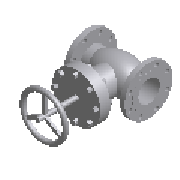
# Autodesk Inventor part: ASME B16.34 Globe Valve Flanged Ends - Class 150 8
Saved by Autodesk Inventor 2019.1 (Build 231200000, 200)
## iProperties
Created: 2018-01-05
Part Number: ASME B16.34 Globe Valve Flanged Ends - Class 150 8
Material: Steel
Description: Globe Valve
Document SubType Name: Modeling
Standard: ASME B16.34
Designer: alid
Standards Organization: ANSI
Language: en-US
Size Designation: 8
Categories: <MemberInstance><Categories><Category DisplayName="Tube &amp; Pipe" InternalName="4347fa0f-2144-441d-94cd-e3e15c92b736" Mnemonic="TUBEANDPIPE"><CategoryParameter DisplayName="Number of Connections" InternalName="04e9c83a-9e20-4a98-a7e1-e8abe87a2846" Mnemonic="NUM_CONNECTIONS"/><CategoryParameter DisplayName="Angles" InternalName="0e0e4fa4-3bd3-4656-a22e-4e07c8c476f8" Mnemonic="ANGLES"><CategoryParameter DisplayName="Angle" InternalName="9188ad83-1b16-48b4-8b0a-76ce729dafa7" Mnemonic="ANGLE"/></CategoryParameter><CategoryParameter DisplayName="SKey" InternalName="3da84699-049a-4bc2-a65a-6696b77c242f" Mnemonic="SKEY"/><CategoryParameter DisplayName="ISOGEN Description" InternalName="7aa3ba45-b821-4467-8584-f9e6f15f2a7d" Mnemonic="ISOGENDESC"/><CategoryParameter DisplayName="ITEM-CODE" InternalName="99cc3b15-24d9-4d38-aac7-792cfbc57acf" Mnemonic="ITEMCODE"/><CategoryParameter DisplayName="NameOfComponent" InternalName="9c74ad13-48a1-45fe-b0f7-5447561f444a" Mnemonic="NAMEOFCOMPONENT"/><CategoryParameter DisplayName="InLineGroups" InternalName="d60be647-bc43-4c18-a13f-9fe4115f8e64" Mnemonic="INLINEGROUPS"/><Category DisplayName="Fittings" InternalName="ed6b26c4-72b8-4f31-9b63-f85ae8f932e4" Mnemonic="FITTINGS"><CategoryParameter DisplayName="Connections" InternalName="dbd721e8-e885-4eea-9011-b5acfd9f61de" Mnemonic="FIT_CONNECTIONS"><CategoryParameter DisplayName="Min Mating Pipe Size" InternalName="11f51b32-3e37-4310-abf7-f1318a1fd129" Mnemonic="MNMPS"/><CategoryParameter DisplayName="MaxEngagement" InternalName="34fdf028-8797-436e-ba07-ca3dee15bd9b" Mnemonic="MAXENGAGEMENT"/><CategoryParameter DisplayName="NominalSize" InternalName="3f94edc7-e459-48db-8f02-8eebf8cffccd" Mnemonic="NS"/><CategoryParameter DisplayName="DisplayName" InternalName="50f521dd-e050-43f7-9895-6b30ea7ed42e" Mnemonic="DISPLAYNAME"/><CategoryParameter DisplayName="Cut Mating Pipe" InternalName="53a63a6e-53d8-4ca9-8880-037731d1cceb" Mnemonic="CMP"/><CategoryParameter DisplayName="Gender Neutral" InternalName="628bd5f1-acad-44e2-9d91-af996ab74fc2" Mnemonic="NEUTRAL"/><CategoryParameter DisplayName="MinEngagement [% of MaxEngagement]" InternalName="7ec1bde5-73f0-45b1-98d8-365a6c67f8ad" Mnemonic="MINENGAGEMENT"/><CategoryParameter DisplayName="Fixed" InternalName="9142902a-6a8a-446d-9eb8-4b7ce7d245ef" Mnemonic="FIXED"/><CategoryParameter DisplayName="Female" InternalName="b366bcb5-a500-4bad-84bb-22f956216d69" Mnemonic="FEMALE"/><CategoryParameter DisplayName="FlipDirection" InternalName="d55dedc0-f14a-4283-86b4-a4eeb253c8aa" Mnemonic="FLIPDIRECTION"/><CategoryParameter DisplayName="ScheduleNumber" InternalName="d6161c62-eb59-4495-a086-874847c10866" Mnemonic="SN"/><CategoryParameter DisplayName="EndTreatment" InternalName="d7f11516-3374-45ca-b1c7-4b2d63244ae2" Mnemonic="ENDTREATMENT"/><CategoryParameter DisplayName="Max Mating Pipe Size" InternalName="e73ef66b-c04b-45ac-9b32-f712653e25ee" Mnemonic="MXMPS"/></CategoryParameter><CategoryParameter DisplayName="Connections" InternalName="dbd721e8-e885-4eea-9011-b5acfd9f61de" Mnemonic="FIT_CONNECTIONS"><CategoryParameter DisplayName="Min Mating Pipe Size" InternalName="11f51b32-3e37-4310-abf7-f1318a1fd129" Mnemonic="MNMPS"/><CategoryParameter DisplayName="MaxEngagement" InternalName="34fdf028-8797-436e-ba07-ca3dee15bd9b" Mnemonic="MAXENGAGEMENT"/><CategoryParameter DisplayName="NominalSize" InternalName="3f94edc7-e459-48db-8f02-8eebf8cffccd" Mnemonic="NS"/><CategoryParameter DisplayName="DisplayName" InternalName="50f521dd-e050-43f7-9895-6b30ea7ed42e" Mnemonic="DISPLAYNAME"/><CategoryParameter DisplayName="Cut Mating Pipe" InternalName="53a63a6e-53d8-4ca9-8880-037731d1cceb" Mnemonic="CMP"/><CategoryParameter DisplayName="Gender Neutral" InternalName="628bd5f1-acad-44e2-9d91-af996ab74fc2" Mnemonic="NEUTRAL"/><CategoryParameter DisplayName="MinEngagement [% of MaxEngagement]" InternalName="7ec1bde5-73f0-45b1-98d8-365a6c67f8ad" Mnemonic="MINENGAGEMENT"/><CategoryParameter DisplayName="Fixed" InternalName="9142902a-6a8a-446d-9eb8-4b7ce7d245ef" Mnemonic="FIXED"/><CategoryParameter DisplayName="Female" InternalName="b366bcb5-a500-4bad-84bb-22f956216d69" Mnemonic="FEMALE"/><CategoryParameter DisplayName="FlipDirection" InternalName="d55dedc0-f14a-4283-86b4-a4eeb253c8aa" Mnemonic="FLIPDIRECTION"/><CategoryParameter DisplayName="ScheduleNumber" InternalName="d6161c62-eb59-4495-a086-874847c10866" Mnemonic="SN"/><CategoryParameter DisplayName="EndTreatment" InternalName="d7f11516-3374-45ca-b1c7-4b2d63244ae2" Mnemonic="ENDTREATMENT"/><CategoryParameter DisplayName="Max Mating Pipe Size" InternalName="e73ef66b-c04b-45ac-9b32-f712653e25ee" Mnemonic="MXMPS"/></CategoryParameter><Category DisplayName="Valves" InternalName="b54f24b4-8c71-4f76-b075-760a31c67e8e" Mnemonic="Valve"><Category DisplayName="Globe Valves" InternalName="921f2858-3697-42bb-925a-27c6a90102c9" Mnemonic="Globe_Valve"/></Category></Category></Category><Category DisplayName="DataType" InternalName="23b78d0f-2648-40c6-8793-ca6db495c9e8" Mnemonic="DATATYPE"><CategoryParameter DisplayName="DisplayName" InternalName="05415f3d-3907-474b-a020-eb9d644f4cf3" Mnemonic="DISPLAYNAME"/><CategoryParameter DisplayName="Standard" InternalName="0c0a119c-1e12-4c84-803f-101930972f5e" Mnemonic="STANDARD"/><CategoryParameter DisplayName="Description" InternalName="13903e3d-64b1-4950-80da-f627842ea37f" Mnemonic="DESCRIPTION"/><CategoryParameter DisplayName="Designation" InternalName="2675968c-4ce5-49e0-a4f5-552d29089031" Mnemonic="DESIGNATION"/><CategoryParameter DisplayName="Default Row" InternalName="2af9ec52-faaa-4026-b378-f9fa4afca842" Mnemonic="DEFAULTROW"/><CategoryParameter DisplayName="Folder Name" InternalName="3f06958e-8713-4116-9be7-ed6184ecc97b" Mnemonic="FOLDERNAME"/><CategoryParameter DisplayName="Revision Guid" InternalName="45a75005-10b1-4dfc-8d6d-dfe629f0b93c" Mnemonic="REVISIONGUID"/><CategoryParameter DisplayName="FileName" InternalName="8b46a4cc-9585-4fed-90c3-899f57e09a73" Mnemonic="FILENAME"/><CategoryParameter DisplayName="StdsOrg" InternalName="8f5914e1-4693-403f-8ab5-d37768198c9d" Mnemonic="STDSORG"/><CategoryParameter DisplayName="Family Version" InternalName="914462f6-6e19-4b14-ba84-155b9680b1d0" Mnemonic="FAMILYREVISION"/><CategoryParameter DisplayName="Standard Revision" InternalName="91d5a463-65c2-4fde-b823-3b7fea5e8e17" Mnemonic="STANDARDREVISION"/><CategoryParameter DisplayName="Member Revision" InternalName="a65d44b9-392f-4f4f-857b-e4b3d54996fe" Mnemonic="MEMBERREVISION"/><CategoryParameter DisplayName="ClipFormat" InternalName="bc51e27b-3422-4e78-93ef-cec197ddf230" Mnemonic="CLIPFORMAT"/><CategoryParameter DisplayName="Manufacturer" InternalName="cd6c7a72-a28a-4e50-99a9-2c7f4e13e5ad" Mnemonic="MANUFACTURER"/><CategoryParameter DisplayName="InternalName" InternalName="cf1d0246-76d9-4b4a-8305-fa0409afb5c1" Mnemonic="INTERNALNAME"/><CategoryParameter DisplayName="IsMetric" InternalName="e2385c5b-1ea4-4823-96a8-8de651266ec3" Mnemonic="ISMETRIC"/><Category DisplayName="Part" InternalName="c0e0b642-3bcb-4cc8-9e80-f96d35c4afa4" Mnemonic="PART"><CategoryParameter DisplayName="Part Number" InternalName="016b6077-bfbe-49bd-92c9-d8d59c39c941" Mnemonic="PARTNUMBER"/><CategoryParameter DisplayName="Stock Number" InternalName="4dba7c1c-e26c-444e-836c-b08b433409a8" Mnemonic="STOCKNUMBER"/><CategoryParameter DisplayName="Material Key" InternalName="5c9a8adb-dd2b-4535-b97f-0a94a95fe41f" Mnemonic="MATERIALKEY"/><CategoryParameter DisplayName="Material" InternalName="818a152a-d3c3-49ca-80ee-df7d91421b8e" Mnemonic="MATERIAL"/></Category></Category><Category DisplayName="LegacyMap" InternalName="dfeab48a-acc2-4514-a11c-1b8dc28c3d5f" Mnemonic="LEGACYMAP"><CategoryParameter DisplayName="CatalogID" InternalName="0da51c36-8fd3-4028-86cc-0c9c9e96136a" Mnemonic="CATALOGID"/><CategoryParameter DisplayName="FamilyID" InternalName="1c0b589c-8bbe-4e1e-80cf-07c0de42ac2a" Mnemonic="FAMILYID"/><CategoryParameter DisplayName="MemberID" InternalName="a368ea03-db8a-4d6e-962b-2aa46306b8f5" Mnemonic="MEMBERID"/></Category></Categories><FamilyTemplate Id="ASME B16.34 Globe Valve Flanged Ends - Class 150"><FamilyTemplateParameters><FamilyTemplateParameter ObjectType="kUserParameterObject" ValueType="xs:double" Id="1" ObjectReferenceKey="A"/><FamilyTemplateParameter ObjectType="kUserParameterObject" ValueType="xs:double" Id="2" ObjectReferenceKey="H"/><FamilyTemplateParameter ObjectType="kUserParameterObject" ValueType="xs:double" Id="3" ObjectReferenceKey="D"/><FamilyTemplateParameter ObjectType="kUserParameterObject" ValueType="xs:double" Id="4" ObjectReferenceKey="t"/><FamilyTemplateParameter ObjectType="kUserParameterObject" ValueType="xs:double" Id="5" ObjectReferenceKey="O"/><FamilyTemplateParameter ObjectType="kUserParameterObject" ValueType="xs:double" Id="6" ObjectReferenceKey="C1"/><FamilyTemplateParameter ObjectType="kUserParameterObject" ValueType="xs:double" Id="7" ObjectReferenceKey="BC"/><FamilyTemplateParameter ObjectType="kUserParameterObject" ValueType="xs:double" Id="8" ObjectReferenceKey="DH"/><FamilyTemplateParameter ObjectType="kUserParameterObject" ValueType="xs:integer" Id="9" ObjectReferenceKey="Nu"/><FamilyTemplateParameter ObjectType="kUserParameterObject" ValueType="xs:double" Id="10" ObjectReferenceKey="R"/><FamilyTemplateParameter ObjectType="kUserParameterObject" ValueType="xs:double" Id="11" ObjectReferenceKey="d"/><FamilyTemplateParameter ObjectType="kUserParameterObject" ValueType="xs:string" Id="120" ObjectReferenceKey="Size_Designation"/><FamilyTemplateParameter ObjectType="kPropertyObject" ValueType="xs:string" Id="100" ObjectReferenceKey="{32853F0F-3444-11d1-9E93-0060B03C1CA6}" SubObjectId="52"/><FamilyTemplateParameter ObjectType="kPropertyObject" ValueType="xs:string" Id="105" ObjectReferenceKey="{32853F0F-3444-11d1-9E93-0060B03C1CA6}" SubObjectId="5"/><FamilyTemplateParameter ObjectType="kPartComponentDefinitionObject" ValueType="xs:string" Id="110" SubObjectId="Material"/></FamilyTemplateParameters></FamilyTemplate><CategoryParameterMap><ParamToTemplateMap><ParamToTemplate CategoryParameter="//CategoryParameter[@InternalName='d60be647-bc43-4c18-a13f-9fe4115f8e64']" ConstantValue="1"/><ParamToTemplate CategoryParameter="//CategoryParameter[@InternalName='04e9c83a-9e20-4a98-a7e1-e8abe87a2846']" ConstantValue="2"/><ParamToTemplate CategoryParameter="//CategoryParameter[@InternalName='0e0e4fa4-3bd3-4656-a22e-4e07c8c476f8']" ConstantValue=""/><ParamToTemplate CategoryParameter="//CategoryParameter[@InternalName='0e0e4fa4-3bd3-4656-a22e-4e07c8c476f8'][1]/CategoryParameter[@InternalName='9188ad83-1b16-48b4-8b0a-76ce729dafa7']" ConstantValue="3.14159265358979"/><ParamToTemplate CategoryParameter="//CategoryParameter[@InternalName='9c74ad13-48a1-45fe-b0f7-5447561f444a']" ConstantValue="VALVE"/><ParamToTemplate CategoryParameter="//CategoryParameter[@InternalName='3da84699-049a-4bc2-a65a-6696b77c242f']" ConstantValue="VGFL"/><ParamToTemplate CategoryParameter="//CategoryParameter[@InternalName='dbd721e8-e885-4eea-9011-b5acfd9f61de'][1]/CategoryParameter[@InternalName='d55dedc0-f14a-4283-86b4-a4eeb253c8aa']" ConstantValue="true"/><ParamToTemplate CategoryParameter="//CategoryParameter[@InternalName='dbd721e8-e885-4eea-9011-b5acfd9f61de'][1]/CategoryParameter[@InternalName='50f521dd-e050-43f7-9895-6b30ea7ed42e']" ConstantValue="Connection1"/><ParamToTemplate CategoryParameter="//CategoryParameter[@InternalName='dbd721e8-e885-4eea-9011-b5acfd9f61de'][1]/CategoryParameter[@InternalName='b366bcb5-a500-4bad-84bb-22f956216d69']" ConstantValue="true"/><ParamToTemplate CategoryParameter="//CategoryParameter[@InternalName='dbd721e8-e885-4eea-9011-b5acfd9f61de'][1]/CategoryParameter[@InternalName='d7f11516-3374-45ca-b1c7-4b2d63244ae2']" ConstantValue="Flanged"/><ParamToTemplate CategoryParameter="//CategoryParameter[@InternalName='dbd721e8-e885-4eea-9011-b5acfd9f61de'][1]/CategoryParameter[@InternalName='9142902a-6a8a-446d-9eb8-4b7ce7d245ef']" ConstantValue="true"/><ParamToTemplate CategoryParameter="//CategoryParameter[@InternalName='dbd721e8-e885-4eea-9011-b5acfd9f61de'][1]/CategoryParameter[@InternalName='34fdf028-8797-436e-ba07-ca3dee15bd9b']" ConstantValue="0"/><ParamToTemplate CategoryParameter="//CategoryParameter[@InternalName='dbd721e8-e885-4eea-9011-b5acfd9f61de'][1]/CategoryParameter[@InternalName='7ec1bde5-73f0-45b1-98d8-365a6c67f8ad']" ConstantValue="0"/><ParamToTemplate CategoryParameter="//CategoryParameter[@InternalName='dbd721e8-e885-4eea-9011-b5acfd9f61de'][2]/CategoryParameter[@InternalName='d55dedc0-f14a-4283-86b4-a4eeb253c8aa']" ConstantValue="false"/><ParamToTemplate CategoryParameter="//CategoryParameter[@InternalName='dbd721e8-e885-4eea-9011-b5acfd9f61de'][2]/CategoryParameter[@InternalName='50f521dd-e050-43f7-9895-6b30ea7ed42e']" ConstantValue="Connection2"/><ParamToTemplate CategoryParameter="//CategoryParameter[@InternalName='dbd721e8-e885-4eea-9011-b5acfd9f61de'][2]/CategoryParameter[@InternalName='b366bcb5-a500-4bad-84bb-22f956216d69']" ConstantValue="true"/><ParamToTemplate CategoryParameter="//CategoryParameter[@InternalName='dbd721e8-e885-4eea-9011-b5acfd9f61de'][2]/CategoryParameter[@InternalName='d7f11516-3374-45ca-b1c7-4b2d63244ae2']" ConstantValue="Flanged"/><ParamToTemplate CategoryParameter="//CategoryParameter[@InternalName='dbd721e8-e885-4eea-9011-b5acfd9f61de'][2]/CategoryParameter[@InternalName='9142902a-6a8a-446d-9eb8-4b7ce7d245ef']" ConstantValue="true"/><ParamToTemplate CategoryParameter="//CategoryParameter[@InternalName='dbd721e8-e885-4eea-9011-b5acfd9f61de'][2]/CategoryParameter[@InternalName='34fdf028-8797-436e-ba07-ca3dee15bd9b']" ConstantValue="0"/><ParamToTemplate CategoryParameter="//CategoryParameter[@InternalName='dbd721e8-e885-4eea-9011-b5acfd9f61de'][2]/CategoryParameter[@InternalName='7ec1bde5-73f0-45b1-98d8-365a6c67f8ad']" ConstantValue="0"/><ParamToTemplate CategoryParameter="//CategoryParameter[@InternalName='dbd721e8-e885-4eea-9011-b5acfd9f61de'][1]/CategoryParameter[@InternalName='628bd5f1-acad-44e2-9d91-af996ab74fc2']" ConstantValue="true"/><ParamToTemplate CategoryParameter="//CategoryParameter[@InternalName='dbd721e8-e885-4eea-9011-b5acfd9f61de'][2]/CategoryParameter[@InternalName='628bd5f1-acad-44e2-9d91-af996ab74fc2']" ConstantValue="true"/><ParamToTemplate CategoryParameter="//CategoryParameter[@InternalName='05415f3d-3907-474b-a020-eb9d644f4cf3']" ConstantValue="ASME B16.34 Globe Valve Flanged Ends - Class 150"/><ParamToTemplate CategoryParameter="//CategoryParameter[@InternalName='cf1d0246-76d9-4b4a-8305-fa0409afb5c1']" ConstantValue="3aee62ce-7efa-48e6-9864-387eb336ef42"/><ParamToTemplate CategoryParameter="//CategoryParameter[@InternalName='3f06958e-8713-4116-9be7-ed6184ecc97b']" ConstantValue="ASME B16.34(42)"/><ParamToTemplate CategoryParameter="//CategoryParameter[@InternalName='914462f6-6e19-4b14-ba84-155b9680b1d0']" ConstantValue="10"/><ParamToTemplate CategoryParameter="//CategoryParameter[@InternalName='13903e3d-64b1-4950-80da-f627842ea37f']" ConstantValue="Globe Valve"/><ParamToTemplate CategoryParameter="//CategoryParameter[@InternalName='8f5914e1-4693-403f-8ab5-d37768198c9d']" ConstantValue="ANSI"/><ParamToTemplate CategoryParameter="//CategoryParameter[@InternalName='0c0a119c-1e12-4c84-803f-101930972f5e']" ConstantValue="ASME B16.34"/><ParamToTemplate CategoryParameter="//CategoryParameter[@InternalName='cd6c7a72-a28a-4e50-99a9-2c7f4e13e5ad']" TemplateParameter="104"/><ParamToTemplate CategoryParameter="//CategoryParameter[@InternalName='91d5a463-65c2-4fde-b823-3b7fea5e8e17']" TemplateParameter="103"/><ParamToTemplate CategoryParameter="//CategoryParameter[@InternalName='bc51e27b-3422-4e78-93ef-cec197ddf230']" ConstantValue="CF_INVENTOR.STDPARTS"/><ParamToTemplate CategoryParameter="//CategoryParameter[@InternalName='e2385c5b-1ea4-4823-96a8-8de651266ec3']" ConstantValue="false"/><ParamToTemplate CategoryParameter="//CategoryParameter[@InternalName='45a75005-10b1-4dfc-8d6d-dfe629f0b93c']" ConstantValue="1603e2bb-d21b-47a1-9595-97303de8b626"/><ParamToTemplate CategoryParameter="//CategoryParameter[@InternalName='2af9ec52-faaa-4026-b378-f9fa4afca842']" ConstantValue="7"/><ParamToTemplate CategoryParameter="//CategoryParameter[@InternalName='0da51c36-8fd3-4028-86cc-0c9c9e96136a']" ConstantValue="4DA64A5D-C2A1-4499-9EC0-0CCCC70B216C"/><ParamToTemplate CategoryParameter="//CategoryParameter[@InternalName='1c0b589c-8bbe-4e1e-80cf-07c0de42ac2a']" ConstantValue="3aee62ce-7efa-48e6-9864-387eb336ef42"/><ParamToTemplate CategoryParameter="//CategoryParameter[@InternalName='99cc3b15-24d9-4d38-aac7-792cfbc57acf']" ConstantValue=""/><ParamToTemplate CategoryParameter="//CategoryParameter[@InternalName='7aa3ba45-b821-4467-8584-f9e6f15f2a7d']" ConstantValue=""/><ParamToTemplate CategoryParameter="//CategoryParameter[@InternalName='dbd721e8-e885-4eea-9011-b5acfd9f61de'][1]/CategoryParameter[@InternalName='3f94edc7-e459-48db-8f02-8eebf8cffccd']" ConstantValue="8"/><ParamToTemplate CategoryParameter="//CategoryParameter[@InternalName='dbd721e8-e885-4eea-9011-b5acfd9f61de'][2]/CategoryParameter[@InternalName='3f94edc7-e459-48db-8f02-8eebf8cffccd']" ConstantValue="8"/><ParamToTemplate CategoryParameter="//CategoryParameter[@InternalName='8b46a4cc-9585-4fed-90c3-899f57e09a73']" ConstantValue="ASME B16.34 Globe Valve Flanged Ends - Class 150 8"/><ParamToTemplate CategoryParameter="//CategoryParameter[@InternalName='a65d44b9-392f-4f4f-857b-e4b3d54996fe']" ConstantValue="e44e4053-20c4-4010-b29f-140cc5881618"/><ParamToTemplate CategoryParameter="//CategoryParameter[@InternalName='a368ea03-db8a-4d6e-962b-2aa46306b8f5']" ConstantValue="8B5BE43C-C9F7-4F65-A638-D02D13F6207C"/><ParamToTemplate CategoryParameter="//CategoryParameter[@InternalName='2675968c-4ce5-49e0-a4f5-552d29089031']" TemplateParameter="100"/><ParamToTemplate CategoryParameter="//CategoryParameter[@InternalName='818a152a-d3c3-49ca-80ee-df7d91421b8e']" TemplateParameter="110"/><ParamToTemplate CategoryParameter="//CategoryParameter[@InternalName='016b6077-bfbe-49bd-92c9-d8d59c39c941']" TemplateParameter="105"/></ParamToTemplateMap></CategoryParameterMap></MemberInstance>
Density: 1 g/cm^3
Appearance: Plate
IsCustomPart: 0
NAME: PIPING: ASME B16.34 Globe Valve Flanged Ends - Class 150
DATA: <meta><inlinegroups number="1" deflen="29.21"></inlinegroups><connections number="2"></connections><angles><a>3.14159265358979</a></angles></meta>
Author: alid
Autodesk Inventor part; units mm, degrees
ref_plane "YZ Plane" through (0, 0, 0) normal (1, 0, 0) x (0, 1, 0)
ref_plane "XZ Plane" through (0, 0, 0) normal (0, 1, 0) x (-1, 0, 0)
sketch "Sketch1" plane through (0, 0, 0) normal (0, 0, 1) x (1, 0, 0)
  line L0 (0, 0) -> (0, 134.874)
  line L1 (0, 134.874) -> (1.524, 134.874)
  line L2 (1.524, 134.874) -> (1.524, 171.45)
  line L3 (1.524, 171.45) -> (28.448, 171.45)
  line L4 (28.448, 171.45) -> (28.448, 109.474)
  line L5 (247.65, 134.874) -> (247.65, 0) construction
  line L6 (495.3, 0) -> (0, 0)
  line L7 (495.3, 0) -> (495.3, 134.874)
  line L8 (495.3, 134.874) -> (493.776, 134.874)
  line L9 (493.776, 134.874) -> (493.776, 171.45)
  line L10 (493.776, 171.45) -> (466.852, 171.45)
  line L11 (466.852, 171.45) -> (466.852, 109.474)
  arc A0 (396.24, 109.474) -> (99.06, 109.474) centre (247.65, -312.4518) ccw
  line L12 (28.448, 109.474) -> (99.06, 109.474)
  line L13 (396.24, 109.474) -> (466.852, 109.474)
  dimension "d0" = 269.748
  dimension "d1" = 342.9
  dimension "d2" = 1.524
  dimension "d3" = 28.448
  dimension "d4" = 495.3
  dimension "d43" = 218.948
  dimension "d44" = 297.18
  constraints: 28 end point, 7 parallel, 7 symmetric about line, 3 point on circle, 2 coincident, 1 centre point, 1 midpoint, 1 perpendicular, 1 point on line, 1 tangent, 1 vertical, 5 other
  measures "d0" diameter of L1 L6
  measures "d1" diameter of L3 L6
  measures "d2" distance of L0.end L1.end
  measures "d3" distance between parallel lines of L4 L0
  measures "d4" distance of L6.start L0.start
  measures "d43" diameter of L12 L6
  measures "d44" distance of L13.start L12.end
revolve "Revolution1" add sketch "Sketch1" angle 360 about axis through (495.3, 0, 0) along (-1, 0, 0)
sketch "Sketch2" plane through (493.776, 0, 0) normal (1, 0, 0) x (0, 0, -1)
  circle A0 centre (0, 0) radius 171.45 projected
  circle A1 centre (0, 0) radius 149.225 construction
  line L0 (0, 0) -> (-137.8659, 57.1059) construction
  circle A2 centre (-137.8659, 57.1059) radius 11.176
  circle A3 centre (0, 0) radius 134.874 projected
  line L1 (-149.225, 0) -> (0, 0) construction
  dimension "d6" = 298.45
  dimension "d8" = 22.352
  dimension "d45" = 22.5
  constraints: 4 end point, 2 centre point, 2 point on circle, 1 coincident, 1 concentric, 1 horizontal
  measures "d6" diameter of A1
  measures "d8" diameter of A2
  measures "d45" angle of L0 L1
extrude "Extrusion1" cut sketch "Sketch2" against normal through all contours A2
pattern_circular "Circular Pattern1" count 8 over 360 about axis through (63.754, 0, 0) along (1, 0, 0) of "Extrusion1"
sketch "Sketch3" plane through (0, 0, 0) normal (0, 1, 0) x (-1, 0, 0)
  line L0 (-495.3, 134.874) -> (-495.3, -134.874) projected
  line L1 (0, 134.874) -> (0, -134.874) projected
  line L2 (-495.3, 0) -> (0, 0) construction
  line L3 (-247.65, 0) -> (-247.65, 623.062)
  line L4 (-247.65, 623.062) -> (-229.8954, 623.062)
  line L5 (-229.8954, 623.062) -> (-229.8954, 578.6755)
  line L6 (-229.8954, 587.5528) -> (-70.104, 587.5528) construction
  arc A0 (-103.2345, 560.9209) -> (-103.2345, 578.6755) centre (-87.8586, 569.7982) ccw
  line L7 (-70.104, 552.0436) -> (-229.8954, 552.0436) construction
  line L8 (-229.8954, 560.9209) -> (-229.8954, 271.018)
  line L9 (-229.8954, 271.018) -> (-76.2, 271.018)
  line L10 (-76.2, 271.018) -> (-76.2, 214.122)
  line L11 (-76.2, 214.122) -> (-127.2286, 214.122)
  line L12 (-127.2286, 214.122) -> (-127.2286, 0)
  line L13 (-247.65, 0) -> (-127.2286, 0)
  line L14 (-70.104, 587.5528) -> (-70.104, 552.0436) construction
  line L15 (-229.8954, 578.6755) -> (-103.2345, 578.6755)
  line L16 (-87.8586, 569.7982) -> (-247.65, 569.7982) construction
  line L17 (-229.8954, 560.9209) -> (-103.2345, 560.9209)
  dimension "d14" = 240.8428
  dimension "d15" = 342.9
  dimension "d16" = 56.896
  dimension "d17" = 214.122
  dimension "d18" = 355.092
  dimension "d19" = 569.7982
  dimension "d20" = 17.7546
  dimension "d21" = 35.5092
  dimension "d22" = 35.5092
  dimension "d23" = 17.7546
  constraints: 33 end point, 6 parallel, 6 perpendicular, 4 point on line, 3 midpoint, 3 tangent, 2 point on circle, 2 symmetric about line, 1 centre point, 1 collinear, 1 other
  measures "d14" diameter of L12 L3
  measures "d15" diameter of L10 L3
  measures "d16" distance between parallel lines of L11 L9
  measures "d17" distance between parallel lines of L13 L11
  measures "d18" diameter of L14 L3
  measures "d19" distance from line of L2 L16.start
  measures "d20" radius of A0
  measures "d21" distance between parallel lines of L6 L4
  measures "d22" diameter of L5 L3
  measures "d23" distance between parallel lines of L17 L15
revolve "Revolution2" add sketch "Sketch3" angle 360 about axis through (247.65, 0, 0) along (0, 0, 1)
sketch "Sketch4" plane through (247.65, 0, 578.6755) normal (0, 0, 1) x (1, 0, 0)
  circle A0 centre (0, 0) radius 144.4155 projected
  arc A1 (130.5649, -61.7142) -> (11.8364, 143.9296) centre (0, 0) ccw
  arc A2 (17.3787, 3.6339) -> (11.8364, 13.2335) centre (0, 0) ccw
  line L0 (0, 0) -> (0, 144.4155) construction
  line L1 (11.8364, 13.2335) -> (11.8364, 143.9296)
  line L2 (17.3787, 3.6339) -> (130.5649, -61.7142)
  circle A3 centre (0, 0) radius 17.7546 projected
  line L3 (0, 0) -> (125.0675, -72.2077) construction
  arc A4 (-11.8364, 143.9296) -> (-130.5649, -61.7142) centre (0, 0) ccw
  arc A5 (-11.8364, 13.2335) -> (-17.3787, 3.6339) centre (0, 0) ccw
  line L4 (-17.3787, 3.6339) -> (-130.5649, -61.7142)
  line L5 (-11.8364, 13.2335) -> (-11.8364, 143.9296)
  arc A6 (-118.7285, -82.2154) -> (118.7285, -82.2154) centre (0, 0) ccw
  arc A7 (-5.5423, -16.8674) -> (5.5423, -16.8674) centre (0, 0) ccw
  line L6 (5.5423, -16.8674) -> (118.7285, -82.2154)
  line L7 (-5.5423, -16.8674) -> (-118.7285, -82.2154)
  point P0 (-125.0675, -72.2077)
  point P1 (0, 144.4155)
  point P2 (125.0675, -72.2077)
  point P3 (-125.0675, -72.2077)
  dimension "d25" = 120
  dimension "d26" = 11.8364
  dimension "d27" = 11.8364
  dimension "d34" = 360
  constraints: 18 point on circle, 16 end point, 6 centre point, 6 concentric, 3 coincident, 2 parallel, 1 vertical, 37 other
  measures "d25" angle of L2 L1
  measures "d26" distance between parallel lines of L0 L1
  measures "d27" distance between parallel lines of L3 L2
extrude "Extrusion2" cut sketch "Sketch4" against normal up to next contours A0 L2 A2 L1 | L5 A3 L4 A0 | A0 L7 A3 L6
sketch "Sketch5" plane through (495.3, 0, 0) normal (1, 0, 0) x (0, 0, -1)
  circle A0 centre (0, 0) radius 134.874 projected
  circle A1 centre (0, 0) radius 101.6
  dimension "d30" = 203.2
  constraints: 1 centre point, 1 coincident, 1 concentric
  measures "d30" diameter of A1
extrude "Extrusion3" cut sketch "Sketch5" against normal through all contours A1
ref_plane "Work Plane1" through (247.65, 0, 292.354) normal (0, 0, 1) x (1, 0, 0)
sketch "Sketch6" plane through (247.65, 0, 292.354) normal (0, 0, 1) x (1, 0, 0)
  circle A0 centre (0, 0) radius 149.225 construction
  line L0 (0, 0) -> (149.225, 0) construction
  circle A1 centre (149.225, 0) radius 13.4112 construction
  line L1 (155.9306, -11.6144) -> (142.5194, -11.6144)
  line L2 (142.5194, -11.6144) -> (135.8138, 0)
  line L3 (135.8138, 0) -> (142.5194, 11.6144)
  line L4 (142.5194, 11.6144) -> (155.9306, 11.6144)
  line L5 (155.9306, 11.6144) -> (162.6362, 0)
  line L6 (162.6362, 0) -> (155.9306, -11.6144)
  circle A2 centre (0, 0) radius 171.45 projected
  dimension "d32" = 298.45
  dimension "d35" = 26.8224
  constraints: 14 end point, 2 coincident, 1 horizontal, 1 horizontal alignment, 1 parallel, 17 other
extrude "Extrusion4" add sketch "Sketch6" against normal blind 99.568 contours L1 L2 L3 L4 L5 L6
pattern_circular "Circular Pattern2" count 8 over 360 about axis through (247.65, 0, 242.57) along (0, 0, -1) of "Extrusion4"
equation "\"d0\" = R"
equation "\"d1\" = O"
equation "\"d3\" = C1"
equation "\"d4\" = A"
equation "\"d43\" = d + 2 * t"
equation "\"d44\" = 0.6 * A"
equation "\"d6\" = BC"
equation "\"d8\" = DH"
equation "\"d14\" = 2.2 * t + 1.1 * d"
equation "\"d15\" = O"
equation "\"d16\" = 2 * C1"
equation "\"d17\" = 0.5 * O + 1.5 * C1"
equation "\"d18\" = D"
equation "\"d19\" = H"
equation "\"d20\" = 0.05 * D"
equation "\"d21\" = 0.1 * D"
equation "\"d22\" = 0.1 * D"
equation "\"d23\" = 0.05 * D"
equation "\"d26\" = 0.0333333 * D"
equation "\"d27\" = 0.0333333 * D"
equation "\"d30\" = d"
equation "\"d32\" = BC"
equation "\"d35\" = 1.2 * DH"
equation "\"d38\" = 3.5 * C1"
equation "\"A\" = 495.3"
equation "\"H\" = 569.7982"
equation "\"D\" = 355.092"
equation "\"d\" = 203.2"
equation "\"t\" = 7.874"
equation "\"O\" = 342.9"
equation "\"C1\" = 28.448"
equation "\"BC\" = 298.45"
equation "\"DH\" = 22.352"
equation "\"R\" = 269.748"
equation "\"d5\" = d + 2 * t"
equation "\"d37\" = 0.75 * C1"
body "Solid1"
